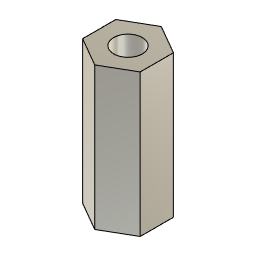
15mmスペーサー (Autodesk Fusion 360 design; units mm, degrees)
Autodesk Fusion 360 part; units mm, degrees
sketch "スケッチ1" plane through (0, 0, 0) normal (0, 0, 1) x (1, 0, 0)
  line L0 (3.5241, 6.0479) -> (-3.4756, 6.076)
  line L1 (-3.4756, 6.076) -> (-6.9997, 0.028)
  line L2 (-6.9997, 0.028) -> (-3.5241, -6.0479)
  line L3 (-3.5241, -6.0479) -> (3.4756, -6.076)
  line L4 (3.4756, -6.076) -> (6.9997, -0.028)
  line L5 (6.9997, -0.028) -> (3.5241, 6.0479)
  circle A0 centre (0, 0) radius 1.5
  line L6 (3.031, 1.7499) -> (0, 3.4999)
  line L7 (0, 3.4999) -> (-3.031, 1.7499)
  line L8 (-3.031, 1.7499) -> (-3.031, -1.7499)
  line L9 (-3.031, -1.7499) -> (0, -3.4999)
  line L10 (0, -3.4999) -> (3.031, -1.7499)
  line L11 (3.031, -1.7499) -> (3.031, 1.7499)
  dimension "d1" = 6.062
  dimension "d2" = 3
  dimension "d3" = 3.031
  constraint coincident A0.centre origin
  measures "d1" distance of A0.centre L5
  measures "d2" diameter of A0
  measures "d3" distance of A0.centre L11
extrude "押し出し1" add sketch "スケッチ1" along normal blind 15 contours L6 L7 L8 L9 L10 L11
